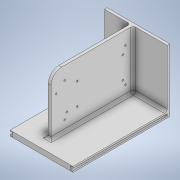
# Autodesk Inventor part: netzteil_halter_unten
Saved by Autodesk Inventor 2021 (Build 250183000, 183)
## iProperties
Created: 2021-11-08
Part Number: netzteil_halter_unten
Material: Generisch
Document SubType Name: Modeling
Designer: Simon
Density: 1 g/cm^3
Appearance: Vorgabe
Author: Simon
Autodesk Inventor part; units mm, degrees
ref_plane "YZ Plane" through (0, 0, 0) normal (1, 0, 0) x (0, 1, 0)
ref_plane "XZ Plane" through (0, 0, 0) normal (0, 1, 0) x (-1, 0, 0)
ref_plane "XY Plane" through (0, 0, 0) normal (0, 0, 1) x (1, 0, 0)
sketch "Skizze1" plane through (0, 0, 0) normal (0, 0, 1) x (1, 0, 0)
  line L0 (-60, 110) -> (60, 110)
  line L1 (60, 110) -> (60, -10)
  line L2 (60, -10) -> (-60, -10)
  line L3 (-60, -10) -> (-60, 110)
  point P0 (0, 0)
  point P1 (0, 110)
  dimension "d0" = 120
  dimension "d1" = 120
  dimension "d2" = 10
  constraints: 8 end point, 2 parallel, 1 horizontal, 1 midpoint, 1 perpendicular, 1 vertical alignment
  measures "d0" distance between parallel lines of L0 L2
  measures "d1" distance between parallel lines of L3 L1
  measures "d2" distance from line of point (0, 0) L2
extrude "Extrusion1" add sketch "Skizze1" against normal blind 5
sketch "Skizze2" plane through (0, 0, 0) normal (0, 0, 1) x (1, 0, 0)
  line L0 (-60, -10) -> (-60, 110) projected
  line L1 (-60, 0) -> (-10.5, 0)
  line L2 (-10.5, 0) -> (-10.5, 110)
  line L3 (-60, 110) -> (60, 110) projected
  line L4 (-5, 110) -> (-5, 0)
  line L5 (-5, 0) -> (60, 0)
  line L6 (-60, -10) -> (60, -10) projected
  line L7 (60, -10) -> (-60, -10) projected
  line L8 (60, 110) -> (60, -10) projected
  line L9 (-10.5, 110) -> (-5, 110)
  line L10 (-60, -10) -> (60, -10)
  line L11 (-60, 0) -> (-60, -3)
  line L12 (-60, -3) -> (-56, -3)
  line L13 (-56, -3) -> (-56, -7)
  line L14 (-56, -7) -> (-60, -7)
  line L15 (-60, -7) -> (-60, -10)
  line L16 (60, -10) -> (60, -7)
  line L17 (60, -7) -> (56, -7)
  line L18 (56, -7) -> (56, -3)
  line L19 (56, -3) -> (60, -3)
  line L20 (60, 0) -> (60, -3)
  point P0 (0, 0)
  dimension "d6" = 5.5
  dimension "d7" = 10
  dimension "d12" = 4
  dimension "d13" = 3
  dimension "d14" = 3
  dimension "d15" = 4
  dimension "d31" = 65
  constraints: 32 end point, 10 point on line, 8 perpendicular, 4 equal length, 3 horizontal, 1 collinear
  measures "d6" distance between parallel lines of L2 L4
  measures "d7" distance between parallel lines of L6 L1
  measures "d12" distance between parallel lines of L12 L14
  measures "d13" distance between parallel lines of L1 L12
  measures "d14" distance between parallel lines of L6 L14
  measures "d15" distance between parallel lines of L0 L13
  measures "d31" distance between parallel lines of L8 L4
extrude "Extrusion2" add sketch "Skizze2" along normal blind 180 contours L0 L14 L13 L12 L1 L2 L3 L4 L5 L8 L19 L18 L17 L6
sketch "Skizze3" plane through (-5, 0, 0) normal (1, 0, 0) x (0, 0, -1)
  line L0 (-131, 85) -> (-15, 85) construction
  line L1 (-15, 85) -> (-15, 20) construction
  line L2 (-15, 20) -> (-131, 20) construction
  line L3 (-131, 20) -> (-131, 85) construction
  line L4 (0, 0) -> (0, 110) projected
  line L5 (0, 0) -> (-180, 0) projected
  line L6 (-107, 72) -> (-20, 72) construction
  line L7 (-20, 72) -> (-20, 30) construction
  line L8 (-20, 30) -> (-107, 30) construction
  line L9 (-107, 30) -> (-107, 72) construction
  line L10 (-147, 71) -> (-127, 71) construction
  line L11 (-127, 71) -> (-127, 31) construction
  line L12 (-127, 31) -> (-147, 31) construction
  line L13 (-147, 31) -> (-147, 71) construction
  dimension "d16" = 116
  dimension "d17" = 65
  dimension "d18" = 15
  dimension "d19" = 20
  dimension "d27" = 87
  dimension "d28" = 42
  dimension "d29" = 5
  dimension "d30" = 10
  dimension "d32" = 20
  dimension "d33" = 40
  dimension "d34" = 20
  dimension "d35" = 11
  constraints: 24 end point, 10 coincident, 6 parallel, 3 horizontal, 3 perpendicular
  measures "d16" distance between parallel lines of L3 L1
  measures "d17" distance of L2.end L0.start
  measures "d18" distance between parallel lines of L4 L1
  measures "d19" distance between parallel lines of L5 L2
  measures "d27" distance between parallel lines of L9 L7
  measures "d28" distance between parallel lines of L8 L6
  measures "d29" distance between parallel lines of L1 L7
  measures "d30" distance between parallel lines of L2 L8
  measures "d32" distance of L10.start L10.end
  measures "d33" distance of L12.end L10.start
  measures "d34" distance between parallel lines of L9 L11
  measures "d35" distance between parallel lines of L2 L12
hole "Bohrung1" at (-5, 85, 131) at (-5, 20, 131) at (-5, 20, 15) at (-5, 85, 15) at (-5, 72, 107) at (-5, 30, 107) at (-5, 30, 20) at (-5, 72, 20) at (-5, 71, 147) at (-5, 31, 127) direction (-1, 0, 0) diameter 3 end through all
sketch "Skizze4" plane through (-5, 0, 0) normal (1, 0, 0) x (0, 0, -1)
  line L0 (0, 110) -> (-180, 110) projected
  line L1 (-156.6453, 110) -> (-156.6453, 0)
  line L2 (0, 0) -> (-180, 0) projected
  line L3 (-156.6453, 0) -> (-180, 0)
  line L4 (-180, 0) -> (-180, 110)
  line L5 (0, -3) -> (-180, -3) projected
  line L6 (-180, 110) -> (-156.6453, 110)
  constraints: 8 end point, 2 collinear, 1 perpendicular, 1 point on line, 1 vertical
extrude "Extrusion3" cut sketch "Skizze4" against normal through all
sketch "Skizze5" plane through (-5, 0, 0) normal (1, 0, 0) x (0, 0, -1)
  point P0 (0, 0)
fillet "Rundung1" radius 20 1 edges at (-7.75, 110, 156.6453)
fillet "Rundung2" radius 1.4 6 edges at (58, -7, 180) (56, -5, 180) (58, -3, 180) (-58, -7, 180) (-56, -5, 180) (-58, -3, 180)
fillet "Rundung3" radius 5 3 edges at (-5, 0, 78.3226) (-10.5, 0, 78.3226) (-7.75, 0, 156.6453)
fillet "Rundung4" radius 5 5 edges at (-3.5355, 1.4645, 0) (-5, 57.5, 0) (-37.75, 0, 0) (-10.5, 57.5, 0) (-11.9645, 1.4645, 0)
equation "\"d13\" = d14"
equation "\"d15\" = d12"
